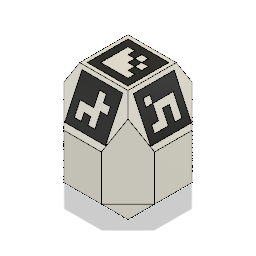
Tracking_die_smaller (Autodesk Fusion 360 design; units mm, degrees)
Autodesk Fusion 360 part; units mm, degrees
note: some values were not read from the file. Set by a fixed rule: which sketch regions a step uses; which face or edge a step refers to.
sketch "Sketch1" plane through (0, 0, 0) normal (0, 1, 0) x (1, 0, 0)
  line L0 (10, -10) -> (-10, -10)
  line L1 (-10, -10) -> (-10, 10)
  line L2 (-10, 10) -> (10, 10)
  line L3 (10, 10) -> (10, -10)
  line L4 (10, -10) -> (-10, 10) construction
  line L5 (-10, -10) -> (10, 10) construction
  dimension "d1" = 20
  dimension "d2" = 20
  constraint perpendicular L0 L1
  constraint parallel L0 L2
  constraint parallel L1 L3
  constraint horizontal L0
  constraint coincident L4 origin
  constraint coincident L5 origin
  measures "d1" distance of L0.end L1.end
  measures "d2" distance of L1.end L2.end
sketch "Sketch3" plane through (0, 0, 0) normal (0, 1, 0) x (1, 0, 0)
  line L0 (10, 10) -> (-10, 10)
  line L1 (-10, 10) -> (-10, -10)
  line L2 (-10, -10) -> (10, -10)
  line L3 (10, -10) -> (10, 10)
  line L4 (10, 10) -> (-10, -10) construction
  line L5 (-10, 10) -> (10, -10) construction
  dimension "d9" = 20
  dimension "d10" = 20
  constraint perpendicular L0 L1
  constraint parallel L0 L2
  constraint parallel L1 L3
  constraint horizontal L0
  constraint coincident L4 origin
  constraint coincident L5 origin
  measures "d9" distance of L1.end L2.end
  measures "d10" distance of L0.end L1.end
extrude "Extrude1" add sketch "Sketch1" along normal blind 10 makes body 1
sketch "Sketch2" plane through (0, 0, 0) normal (0, 1, 0) x (1, 0, 0)
  line L0 (14.1421, 0) -> (0, -14.1421)
  line L1 (0, -14.1421) -> (-14.1421, 0)
  line L2 (-14.1421, 0) -> (0, 14.1421)
  line L3 (0, 14.1421) -> (14.1421, 0)
  line L4 (14.1421, 0) -> (-14.1421, 0) construction
  line L5 (0, -14.1421) -> (0, 14.1421) construction
  dimension "d5" = 20
  dimension "d6" = 20
  constraint perpendicular L0 L1
  constraint parallel L0 L2
  constraint parallel L1 L3
  constraint coincident L4 origin
  constraint coincident L5 origin
  measures "d5" distance of L1.end L2.end
  measures "d6" distance of L0.end L1.end
sketch "Sketch4" plane through (0, 10, 0) normal (0, 1, 0) x (-1, 0, 0)
  line L0 (-10, -10) -> (10, -10)
  line L1 (10, -10) -> (10, 10)
  line L2 (10, 10) -> (-10, 10)
  line L3 (-10, 10) -> (-10, -10)
  line L4 (-10, -10) -> (10, -10)
  line L5 (10, -10) -> (10, 10)
  line L6 (10, 10) -> (-10, 10)
  line L7 (-10, 10) -> (-10, -10)
  line L8 (-10, -10) -> (10, 10) construction
  line L9 (10, -10) -> (-10, 10) construction
  dimension "d11" = 20
  dimension "d12" = 20
  constraint perpendicular L4 L5
  constraint parallel L4 L6
  constraint parallel L5 L7
  constraint horizontal L4
  constraint coincident L8 origin
  constraint coincident L9 origin
  measures "d11" distance of L1.end L2.end
  measures "d12" distance of L0.end L1.end
extrude "Extrude3" add sketch "Sketch4" along normal blind 10 draft -25 bodies 1
move_body "Move1" bodies 1 to x (1, 0, 0) y (0, 1, 0) z (0, 0, 1) at (0, 5, 0)
sketch "Sketch5" plane through (0, 5, 0) normal (0, -1, 0) x (1, 0, 0)
  line L0 (-10, -10) -> (10, -10)
  line L1 (10, -10) -> (10, 10)
  line L2 (10, 10) -> (-10, 10)
  line L3 (-10, 10) -> (-10, -10)
  line L4 (10, -10) -> (-10, -10)
  line L5 (-10, -10) -> (-10, 10)
  line L6 (-10, 10) -> (10, 10)
  line L7 (10, 10) -> (10, -10)
  line L8 (10, -10) -> (-10, 10) construction
  line L9 (-10, -10) -> (10, 10) construction
  dimension "d15" = 20
  dimension "d16" = 20
  constraint perpendicular L4 L5
  constraint parallel L4 L6
  constraint parallel L5 L7
  constraint horizontal L4
  constraint coincident L8 origin
  constraint coincident L9 origin
  measures "d15" distance of L2.end L1.end
  measures "d16" distance of L0.start L2.end
extrude "Extrude4" add sketch "Sketch3" against normal blind 5 draft -45 separate body makes body 2
move_body "Move2" bodies 1 to x (1, 0, 0) y (0, 1, 0) z (0, 0, 1) at (0, -5, 0)
sketch "Sketch6" plane through (0, 20, 0) normal (0, 1, 0) x (-1, 0, 0)
  line L0 (5.3369, 5.3369) -> (-5.3369, 5.3369)
  line L1 (-5.3369, 5.3369) -> (-5.3369, -5.3369)
  line L2 (-5.3369, -5.3369) -> (5.3369, -5.3369)
  line L3 (5.3369, -5.3369) -> (5.3369, 5.3369)
  line L4 (-14.1421, 0) -> (0, 14.1421)
  line L5 (0, 14.1421) -> (14.1421, 0)
  line L6 (14.1421, 0) -> (0, -14.1421)
  line L7 (0, -14.1421) -> (-14.1421, 0)
  line L8 (-14.1421, 0) -> (14.1421, 0) construction
  line L9 (0, 14.1421) -> (0, -14.1421) construction
  line L10 (-15.1463, -15.1463) -> (15.1463, -15.1463)
  line L11 (15.1463, -15.1463) -> (15.1463, 15.1463)
  line L12 (15.1463, 15.1463) -> (-15.1463, 15.1463)
  line L13 (-15.1463, 15.1463) -> (-15.1463, -15.1463)
  line L14 (-15.1463, -15.1463) -> (15.1463, 15.1463) construction
  line L15 (15.1463, -15.1463) -> (-15.1463, 15.1463) construction
  dimension "d19" = 20
  dimension "d20" = 20
  constraint perpendicular L4 L5
  constraint parallel L4 L6
  constraint parallel L5 L7
  constraint coincident L8 origin
  constraint coincident L9 origin
  constraint perpendicular L10 L11
  constraint parallel L10 L12
  constraint parallel L11 L13
  constraint horizontal L10
  constraint coincident L14 origin
  constraint coincident L15 origin
  measures "d19" distance of L5.end L6.end
  measures "d20" distance of L4.end L5.end
extrude "Extrude5" cut sketch "Sketch6" against normal blind 25 contours L10 L11 L12 L13 bodies 1 2
sketch "Sketch23" plane through (0, -5, 0) normal (0, -1, 0) x (1, 0, 0)
  line L0 (-5, -5) -> (5, -5)
  line L1 (5, -5) -> (5, 5)
  line L2 (5, 5) -> (-5, 5)
  line L3 (-5, 5) -> (-5, -5)
  line L4 (3.5183, 5.5393) -> (-5.5622, -3.482)
  line L5 (-5.5622, -3.482) -> (-3.5183, -5.5393)
  line L6 (-3.5183, -5.5393) -> (5.5622, 3.482)
  line L7 (5.5622, 3.482) -> (3.5183, 5.5393)
  line L8 (3.5183, 5.5393) -> (-3.5183, -5.5393) construction
  line L9 (-5.5622, -3.482) -> (5.5622, 3.482) construction
  dimension "d418" = 12.8
  dimension "d419" = 2.9
  constraint perpendicular L4 L5
  constraint parallel L4 L6
  constraint parallel L5 L7
  constraint coincident L8 origin
  constraint coincident L9 origin
  measures "d418" distance of L5.end L6.end
  measures "d419" distance of L4.end L5.end
sketch "Sketch8" plane through (-12.0442, 5.6163, 0) normal (-0.906308, 0.422618, 0) x (0, 0, 1)
  line L0 (4.1421, 4.8369) -> (7.0711, 11.7673)
  line L1 (7.0711, 11.7673) -> (5.3369, 15.8707)
  line L2 (5.3369, 15.8707) -> (-5.3369, 15.8707)
  line L3 (-5.3369, 15.8707) -> (-7.0711, 11.7673)
  line L4 (-7.0711, 11.7673) -> (-4.1421, 4.8369)
  line L5 (-4.1421, 4.8369) -> (4.1421, 4.8369)
  line L6 (-4.5277, 15.1063) -> (4.4723, 15.1063)
  line L7 (4.4723, 15.1063) -> (4.4723, 6.1063)
  line L8 (4.4723, 6.1063) -> (-4.5277, 6.1063)
  line L9 (-4.5277, 6.1063) -> (-4.5277, 15.1063)
  line L10 (-4.5277, 13.6063) -> (-4.5277, 12.1063)
  line L11 (-4.5277, 12.1063) -> (-4.5277, 10.6063)
  line L12 (-4.5277, 10.6063) -> (-4.5437, 9.1064)
  line L13 (-4.5437, 9.1064) -> (-4.553, 7.6064)
  line L14 (-4.553, 7.6064) -> (-4.5277, 6.1063)
  line L15 (-3.0277, 15.1063) -> (-1.5277, 15.1063)
  line L16 (-1.5277, 15.1063) -> (-0.0277, 15.1063)
  line L17 (-0.0277, 15.1063) -> (1.4723, 15.1063)
  line L18 (1.4723, 15.1063) -> (2.9723, 15.1063)
  line L19 (2.9814, 13.6063) -> (1.4814, 13.6063)
  line L20 (1.4814, 13.6063) -> (1.4814, 12.1063)
  line L21 (1.4814, 12.1063) -> (2.9814, 12.1063)
  line L22 (2.9814, 12.1063) -> (2.9814, 13.6063)
  line L23 (1.4814, 12.1063) -> (-0.0186, 12.1063)
  line L24 (-0.0186, 12.1063) -> (-0.0186, 10.6063)
  line L25 (-0.0186, 10.6063) -> (1.4814, 10.6063)
  line L26 (1.4814, 10.6063) -> (1.4814, 12.1063)
  line L27 (1.4814, 10.6063) -> (1.4814, 9.1063)
  line L28 (1.4814, 10.6063) -> (2.9814, 10.6063)
  line L29 (2.9814, 10.6063) -> (2.9814, 7.6063)
  line L30 (2.9814, 7.6063) -> (-1.5186, 7.6063)
  line L31 (-1.5186, 7.6063) -> (-1.5186, 9.1063)
  line L32 (1.4814, 9.1063) -> (-0.0186, 9.1063)
  line L33 (-0.0186, 9.1063) -> (-0.0186, 10.6063)
  line L34 (-0.0186, 10.6063) -> (-3.0186, 10.6063)
  line L35 (-3.0186, 10.6063) -> (-3.0186, 9.1063)
  line L36 (-3.0186, 9.1063) -> (-1.5186, 9.1063)
  dimension "d27" = 9
  dimension "d28" = 9
  dimension "d31" = 1.5
  dimension "d32" = 1.5
  dimension "d33" = 1.5
  dimension "d34" = 1.5
  dimension "d35" = 1.5
  dimension "d36" = 1.5
  dimension "d37" = 1.5
  dimension "d38" = 1.5
  dimension "d317" = 1.5
  dimension "d318" = 1.5
  dimension "d319" = 1.5
  dimension "d320" = 1.5
  dimension "d329" = 1.5
  dimension "d330" = 1.5
  dimension "d331" = 3
  dimension "d332" = 4.5
  dimension "d333" = 1.5
  dimension "d334" = 1.5
  dimension "d335" = 3
  dimension "d336" = 1.5
  constraint horizontal L6
  constraint vertical L7
  constraint horizontal L8
  constraint vertical L9
  constraint coincident L9 L10.start
  constraint coincident L6 L15.start
  constraint midpoint L9 L11.end
  constraint parallel L6 L16
  constraint parallel L6 L17
  constraint parallel L6 L18
  constraint horizontal L19
  constraint vertical L20
  constraint horizontal L21
  constraint vertical L22
  constraint horizontal L23
  constraint vertical L24
  constraint horizontal L25
  constraint vertical L26
  constraint perpendicular L25 L27
  constraint perpendicular L27 L28
  constraint perpendicular L28 L29
  constraint perpendicular L29 L30
  constraint perpendicular L30 L31
  constraint perpendicular L27 L32
  constraint perpendicular L24 L34
  constraint perpendicular L34 L35
  measures "d27" distance of L6.start L6.end
  measures "d28" distance of L6.start L8.end
  measures "d31" distance of L10.start L10.end
  measures "d32" distance of L10.end L11.end
  measures "d33" distance of L11.end L12.end
  measures "d34" distance of L12.end L13.end
  measures "d35" distance of L15.start L15.end
  measures "d36" distance of L15.end L16.end
  measures "d37" distance of L16.end L17.end
  measures "d38" distance of L17.end L18.end
  measures "d317" distance of L19.start L19.end
  measures "d318" distance of L19.start L21.end
  measures "d319" distance of L20.end L23.end
  measures "d320" distance of L20.end L25.end
  measures "d329" distance of L25.end L27.end
  measures "d330" distance of L25.end L28.end
  measures "d331" distance of L28.end L29.end
  measures "d332" distance of L29.end L30.end
  measures "d333" distance of L30.end L31.end
  measures "d334" distance of L27.end L32.end
  measures "d335" distance of L24.end L34.end
  measures "d336" distance of L34.end L35.end
sketch "Sketch13" plane through (0, 5.6163, -12.0442) normal (0, 0.422618, -0.906308) x (-1, 0, 0)
  line L0 (-7.0711, 11.7673) -> (-4.1421, 4.8369)
  line L1 (-4.1421, 4.8369) -> (4.1421, 4.8369)
  line L2 (4.1421, 4.8369) -> (7.0711, 11.7673)
  line L3 (7.0711, 11.7673) -> (5.3369, 15.8707)
  line L4 (5.3369, 15.8707) -> (-5.3369, 15.8707)
  line L5 (-5.3369, 15.8707) -> (-7.0711, 11.7673)
  line L6 (-4.5, 15) -> (4.5, 15)
  line L7 (4.5, 15) -> (4.5, 6)
  line L8 (4.5, 6) -> (-4.5, 6)
  line L9 (-4.5, 6) -> (-4.5, 15)
  line L10 (-4.5, 15) -> (-4.5, 13.5)
  line L11 (-4.5, 13.5) -> (-4.5, 12)
  line L12 (-4.5, 12) -> (-4.5, 10.5)
  line L13 (-4.5, 10.5) -> (-4.5, 12)
  line L14 (-4.5, 12) -> (-4.5, 10.5)
  line L15 (-4.5, 6) -> (-4.5, 10.5)
  line L16 (-4.5, 15) -> (-3, 15)
  line L17 (-3, 15) -> (-1.5, 15)
  line L18 (-1.5, 15) -> (0, 15)
  line L19 (0, 15) -> (1.5, 15)
  line L20 (1.5, 15) -> (3, 15)
  line L21 (-3, 7.5) -> (-3, 10.5)
  line L22 (-3, 10.5) -> (-1.5, 10.5)
  line L23 (-1.5, 10.5) -> (-1.5, 9)
  line L24 (-1.5, 9) -> (1.5, 9)
  line L25 (1.5, 9) -> (1.5, 10.5)
  line L26 (3, 10.5) -> (3, 9)
  line L27 (3, 9) -> (1.5, 9)
  line L28 (1.5, 9) -> (1.5, 7.5)
  line L29 (1.5, 12) -> (3, 12)
  line L30 (1.5, 12) -> (1.5, 13.5)
  line L31 (3, 12) -> (3, 13.5)
  line L32 (1.5, 13.5) -> (3, 13.5)
  line L33 (-3, 7.5) -> (1.5, 7.5)
  line L34 (-1.5, 10.5) -> (0, 10.5)
  line L35 (0, 10.5) -> (0, 12)
  line L36 (-1.5, 10.5) -> (-1.5, 13.5)
  line L37 (0, 10.5) -> (0, 13.5)
  line L38 (-1.5, 13.5) -> (0, 13.5)
  line L39 (1.5, 10.5) -> (3, 10.5)
  dimension "d39" = 9
  dimension "d40" = 9
  dimension "d41" = 1.5
  dimension "d42" = 1.5
  dimension "d43" = 1.5
  dimension "d44" = 1.5
  dimension "d45" = 1.5
  dimension "d46" = 1.5
  dimension "d47" = 1.5
  dimension "d48" = 1.5
  dimension "d49" = 1.5
  dimension "d341" = 3
  dimension "d342" = 1.5
  dimension "d343" = 1.5
  dimension "d344" = 3
  dimension "d345" = 1.5
  dimension "d346" = 3
  dimension "d347" = 3
  constraint horizontal L6
  constraint vertical L7
  constraint horizontal L8
  constraint vertical L9
  constraint coincident L6 L16.end
  constraint perpendicular L6 L10
  constraint coincident L9 L11.end
  constraint midpoint L9 L12.end
  constraint parallel L9 L14
  constraint midpoint L6 L18.end
  constraint parallel L6 L19
  constraint coincident L6 L20.end
  constraint perpendicular L21 L22
  constraint perpendicular L22 L23
  constraint perpendicular L23 L24
  constraint perpendicular L24 L25
  constraint perpendicular L28 L33
  constraint perpendicular L23 L34
  constraint perpendicular L22 L35
  constraint perpendicular L34 L36
  constraint perpendicular L34 L37
  constraint perpendicular L37 L38
  constraint perpendicular L26 L39
  measures "d39" distance of L6.start L6.end
  measures "d40" distance of L6.start L8.end
  measures "d41" distance of L6.start L10.end
  measures "d42" distance of L10.end L11.end
  measures "d43" distance of L11.end L12.end
  measures "d44" distance of L12.end L11.end
  measures "d45" distance of L11.end L12.end
  measures "d46" distance of L16.end L17.end
  measures "d47" distance of L17.end L18.end
  measures "d48" distance of L18.end L19.end
  measures "d49" distance of L19.end L20.end
  measures "d341" distance of L21.start L21.end
  measures "d342" distance of L21.end L22.end
  measures "d343" distance of L22.end L23.end
  measures "d344" distance of L23.end L24.end
  measures "d345" distance of L24.end L25.end
  measures "d346" distance of L22.end L36.end
  measures "d347" distance of L34.end L37.end
sketch "Sketch14" plane through (12.0442, 5.6163, 0) normal (0.906308, 0.422618, 0) x (0, 0, -1)
  line L0 (4.1421, 4.8369) -> (7.0711, 11.7673)
  line L1 (7.0711, 11.7673) -> (5.3369, 15.8707)
  line L2 (5.3369, 15.8707) -> (-5.3369, 15.8707)
  line L3 (-5.3369, 15.8707) -> (-7.0711, 11.7673)
  line L4 (-7.0711, 11.7673) -> (-4.1421, 4.8369)
  line L5 (-4.1421, 4.8369) -> (4.1421, 4.8369)
  line L6 (-4.5281, 14.9652) -> (4.4719, 14.9652)
  line L7 (4.4719, 14.9652) -> (4.4719, 5.9652)
  line L8 (4.4719, 5.9652) -> (-4.5281, 5.9652)
  line L9 (-4.5281, 5.9652) -> (-4.5281, 14.9652)
  line L10 (-4.5281, 14.9652) -> (-3.0281, 14.9652)
  line L11 (-3.0281, 14.9652) -> (-1.5281, 14.9652)
  line L12 (-1.5281, 14.9652) -> (-0.0281, 14.9652)
  line L13 (-0.0281, 14.9652) -> (1.4719, 14.9652)
  line L14 (1.4719, 14.9652) -> (2.9719, 14.9652)
  line L15 (-4.5281, 14.9652) -> (-4.5281, 13.4566)
  line L16 (-4.5281, 14.9652) -> (-4.5281, 13.4652)
  line L17 (-4.5281, 13.4566) -> (-4.5281, 11.9566)
  line L18 (-4.5281, 11.9566) -> (-4.5281, 10.4566)
  line L19 (-4.5281, 10.4566) -> (-4.5281, 8.9566)
  line L20 (-4.5281, 8.9566) -> (-4.5281, 7.4566)
  line L21 (-3.0281, 7.4566) -> (-0.0281, 7.4566)
  line L22 (-0.0281, 7.4566) -> (-0.0281, 10.4566)
  line L23 (-0.0281, 10.4566) -> (1.4719, 10.4566)
  line L24 (1.4719, 10.4566) -> (1.4719, 7.4566)
  line L25 (1.4719, 7.4566) -> (2.9719, 7.4566)
  line L26 (2.9719, 7.4566) -> (2.9719, 11.9566)
  line L27 (2.9719, 11.9566) -> (-1.5281, 11.9566)
  line L28 (-1.5281, 11.9566) -> (-1.5281, 8.9566)
  line L29 (-1.5281, 8.9566) -> (-3.0281, 8.9566)
  line L30 (-3.0281, 8.9566) -> (-3.0281, 7.4566)
  line L31 (-1.5281, 11.9566) -> (-1.5281, 13.4566)
  line L32 (-1.5281, 13.4566) -> (-3.0281, 13.4566)
  line L33 (-3.0281, 13.4566) -> (-3.0281, 11.9566)
  line L34 (-3.0281, 11.9566) -> (-1.5281, 11.9566)
  dimension "d50" = 9
  dimension "d51" = 9
  dimension "d52" = 1.5
  dimension "d53" = 1.5
  dimension "d54" = 1.5
  dimension "d55" = 1.5
  dimension "d56" = 1.5
  dimension "d57" = 1.5
  dimension "d58" = 1.5
  dimension "d59" = 1.5
  dimension "d60" = 1.5
  dimension "d61" = 1.5
  dimension "d352" = 3
  dimension "d353" = 3
  dimension "d354" = 1.5
  dimension "d355" = 1.5
  dimension "d356" = 4.5
  dimension "d357" = 4.5
  dimension "d358" = 3
  dimension "d359" = 1.5
  dimension "d360" = 1.5
  dimension "d361" = 1.5
  dimension "d362" = 1.5
  dimension "d363" = 1.5
  constraint horizontal L6
  constraint vertical L7
  constraint horizontal L8
  constraint vertical L9
  constraint perpendicular L9 L10
  constraint perpendicular L9 L11
  constraint parallel L6 L12
  constraint parallel L6 L13
  constraint parallel L6 L14
  constraint coincident L9 L15.end
  constraint perpendicular L6 L16
  constraint parallel L9 L17
  constraint parallel L9 L18
  constraint parallel L9 L19
  constraint parallel L9 L20
  constraint perpendicular L22 L23
  constraint perpendicular L25 L26
  constraint perpendicular L26 L27
  constraint perpendicular L27 L28
  constraint perpendicular L28 L29
  constraint perpendicular L21 L30
  constraint perpendicular L27 L31
  constraint perpendicular L31 L32
  constraint perpendicular L32 L33
  measures "d50" distance of L6.start L6.end
  measures "d51" distance of L6.start L8.end
  measures "d52" distance of L6.start L10.end
  measures "d53" distance of L10.end L11.end
  measures "d54" distance of L11.end L12.end
  measures "d55" distance of L12.end L13.end
  measures "d56" distance of L13.end L14.end
  measures "d57" distance of L6.start L16.end
  measures "d58" distance of L15.end L17.end
  measures "d59" distance of L17.end L18.end
  measures "d60" distance of L18.end L19.end
  measures "d61" distance of L19.end L20.end
  measures "d352" distance of L21.start L21.end
  measures "d353" distance of L21.end L22.end
  measures "d354" distance of L22.end L23.end
  measures "d355" distance of L24.end L25.end
  measures "d356" distance of L25.end L26.end
  measures "d357" distance of L26.end L27.end
  measures "d358" distance of L27.end L28.end
  measures "d359" distance of L28.end L29.end
  measures "d360" distance of L29.end L21.start
  measures "d361" distance of L27.end L31.end
  measures "d362" distance of L31.end L32.end
  measures "d363" distance of L32.end L33.end
sketch "Sketch15" plane through (0, 5.6163, 12.0442) normal (0, 0.422618, 0.906308) x (1, 0, 0)
  line L0 (4.1421, 4.8369) -> (7.0711, 11.7673)
  line L1 (7.0711, 11.7673) -> (5.3369, 15.8707)
  line L2 (5.3369, 15.8707) -> (-5.3369, 15.8707)
  line L3 (-5.3369, 15.8707) -> (-7.0711, 11.7673)
  line L4 (-7.0711, 11.7673) -> (-4.1421, 4.8369)
  line L5 (-4.1421, 4.8369) -> (4.1421, 4.8369)
  line L6 (-4.4601, 15.0583) -> (4.5399, 15.0583)
  line L7 (4.5399, 15.0583) -> (4.5399, 6.0583)
  line L8 (4.5399, 6.0583) -> (-4.4601, 6.0583)
  line L9 (-4.4601, 6.0583) -> (-4.4601, 15.0583)
  line L10 (-4.4601, 15.0583) -> (-2.9601, 15.0583)
  line L11 (-2.9601, 15.0583) -> (-1.3135, 15.0583)
  line L12 (-2.9601, 15.0583) -> (-1.4601, 15.0583)
  line L13 (-1.4601, 15.0583) -> (0.0399, 15.0583)
  line L14 (0.0399, 15.0583) -> (1.5399, 15.0583)
  line L15 (1.5399, 15.0583) -> (3.0399, 15.0583)
  line L16 (-4.4601, 15.0583) -> (-4.4601, 13.5583)
  line L17 (-4.4601, 13.5583) -> (-4.4601, 12.0583)
  line L18 (-4.4601, 12.0583) -> (-4.4601, 10.5583)
  line L19 (-4.4601, 10.5583) -> (-4.4601, 9.0583)
  line L20 (-4.4601, 9.0583) -> (-4.4601, 7.5583)
  line L21 (-2.9601, 7.5583) -> (-1.4601, 7.5583)
  line L22 (-2.9601, 7.5583) -> (-2.9601, 10.5583)
  line L23 (-2.9601, 10.5583) -> (0.0399, 10.5583)
  line L24 (-1.4601, 7.5583) -> (-1.4601, 9.0583)
  line L25 (-1.4601, 9.0583) -> (0.0399, 9.0583)
  line L26 (0.0399, 9.0583) -> (0.0399, 7.5583)
  line L27 (0.0399, 7.5583) -> (1.5399, 7.5583)
  line L28 (1.5399, 7.5583) -> (1.5399, 10.5583)
  line L29 (1.5399, 10.5583) -> (3.0399, 10.5583)
  line L30 (3.0399, 10.5583) -> (3.0399, 12.0583)
  line L31 (3.0399, 12.0583) -> (1.5399, 12.0583)
  line L32 (1.5399, 12.0583) -> (1.5399, 13.5583)
  line L33 (1.5399, 13.5583) -> (0.0399, 13.5583)
  line L34 (0.0399, 13.5583) -> (0.0399, 10.5583)
  dimension "d62" = 9
  dimension "d63" = 9
  dimension "d64" = 1.5
  dimension "d65" = 1.5
  dimension "d66" = 1.5
  dimension "d67" = 1.5
  dimension "d68" = 1.5
  dimension "d69" = 1.5
  dimension "d70" = 1.5
  dimension "d71" = 1.5
  dimension "d72" = 1.5
  dimension "d73" = 1.5
  dimension "d368" = 1.5
  dimension "d369" = 3
  dimension "d370" = 3
  dimension "d371" = 1.5
  dimension "d372" = 1.5
  dimension "d373" = 1.5
  dimension "d374" = 3
  dimension "d375" = 1.5
  dimension "d376" = 1.5
  dimension "d377" = 1.5
  dimension "d378" = 1.5
  dimension "d379" = 1.5
  dimension "d380" = 3
  constraint horizontal L6
  constraint vertical L7
  constraint horizontal L8
  constraint vertical L9
  constraint perpendicular L9 L10
  constraint coincident L6 L11.end
  constraint parallel L6 L12
  constraint midpoint L6 L13.end
  constraint parallel L6 L14
  constraint parallel L6 L15
  constraint perpendicular L10 L16
  constraint parallel L9 L17
  constraint parallel L9 L18
  constraint parallel L9 L19
  constraint parallel L9 L20
  constraint perpendicular L24 L25
  constraint perpendicular L25 L26
  constraint perpendicular L24 L27
  constraint perpendicular L27 L28
  constraint perpendicular L28 L29
  constraint perpendicular L29 L30
  constraint perpendicular L30 L31
  constraint perpendicular L32 L33
  measures "d62" distance of L6.start L6.end
  measures "d63" distance of L6.start L8.end
  measures "d64" distance of L6.start L10.end
  measures "d65" distance of L10.end L12.end
  measures "d66" distance of L12.end L13.end
  measures "d67" distance of L13.end L14.end
  measures "d68" distance of L14.end L15.end
  measures "d69" distance of L6.start L16.end
  measures "d70" distance of L16.end L17.end
  measures "d71" distance of L17.end L18.end
  measures "d72" distance of L18.end L19.end
  measures "d73" distance of L19.end L20.end
  measures "d368" distance of L21.start L21.end
  measures "d369" distance of L21.start L22.end
  measures "d370" distance of L22.end L23.end
  measures "d371" distance of L21.end L24.end
  measures "d372" distance of L24.end L25.end
  measures "d373" distance of L26.end L27.end
  measures "d374" distance of L27.end L28.end
  measures "d375" distance of L28.end L29.end
  measures "d376" distance of L29.end L30.end
  measures "d377" distance of L30.end L31.end
  measures "d378" distance of L31.end L32.end
  measures "d379" distance of L32.end L33.end
  measures "d380" distance of L33.end L23.end
sketch "Sketch16" plane through (0, 20, 0) normal (0, 1, 0) x (-1, 0, 0)
  line L0 (5.3369, 5.3369) -> (-5.3369, 5.3369)
  line L1 (-5.3369, 5.3369) -> (-5.3369, -5.3369)
  line L2 (-5.3369, -5.3369) -> (5.3369, -5.3369)
  line L3 (5.3369, -5.3369) -> (5.3369, 5.3369)
  line L4 (4.5, -4.5) -> (-4.5, -4.5)
  line L5 (-4.5, -4.5) -> (-4.5, 4.5)
  line L6 (-4.5, 4.5) -> (4.5, 4.5)
  line L7 (4.5, 4.5) -> (4.5, -4.5)
  line L8 (4.5, -4.5) -> (3, -4.5)
  line L9 (4.5, -4.5) -> (4.5, -3)
  line L10 (4.5, -3) -> (4.5, -1.5)
  line L11 (4.5, -1.5) -> (4.5, 0)
  line L12 (4.5, 0) -> (4.5, 1.6193)
  line L13 (4.5, 0) -> (4.5, 1.5)
  line L14 (4.5, 1.5) -> (4.5, 3)
  line L15 (4.5, -4.5) -> (3, -4.5)
  line L16 (3, -4.5) -> (1.5, -4.5)
  line L17 (1.5, -4.5) -> (0, -4.5)
  line L18 (0, -4.5) -> (-1.5, -4.5)
  line L19 (-1.5, -4.5) -> (-3, -4.5)
  line L20 (-3, -4.5) -> (-1.5, -4.5)
  line L21 (3, -3) -> (1.5, -3)
  line L22 (1.5, -3) -> (1.5, -1.5)
  line L23 (1.5, -1.5) -> (0, -1.5)
  line L24 (0, -1.5) -> (0, 0)
  line L25 (0, -1.5) -> (0, -3)
  line L26 (0, -1.5) -> (-1.5, -1.5)
  line L27 (-1.5, -1.5) -> (-1.5, -3)
  line L28 (-1.5, -3) -> (0, -3)
  line L29 (3, -3) -> (3, 3)
  line L30 (3, 3) -> (-3, 3)
  line L31 (-3, 3) -> (-3, 1.5)
  line L32 (-3, 1.5) -> (-1.5, 1.5)
  line L33 (-1.5, 1.5) -> (-1.5, 0)
  line L34 (-1.5, 0) -> (0, 0)
  line L35 (-1.5, -1.5) -> (-1.5, 0)
  line L36 (-1.5, 0) -> (-3, 0)
  line L37 (-3, 0) -> (-3, -1.5)
  line L38 (-3, -1.5) -> (-1.5, -1.5)
  dimension "d74" = 9
  dimension "d75" = 9
  dimension "d76" = 1.5
  dimension "d77" = 1.5
  dimension "d78" = 1.5
  dimension "d79" = 1.5
  dimension "d80" = 1.5
  dimension "d81" = 1.5
  dimension "d82" = 1.5
  dimension "d83" = 1.5
  dimension "d84" = 1.5
  dimension "d85" = 1.5
  dimension "d385" = 1.5
  dimension "d386" = 1.5
  dimension "d387" = 1.5
  dimension "d388" = 1.5
  dimension "d392" = 6
  dimension "d393" = 6
  dimension "d394" = 1.5
  dimension "d395" = 1.5
  dimension "d396" = 1.5
  dimension "d397" = 1.5
  dimension "d398" = 1.5
  constraint perpendicular L4 L5
  constraint parallel L4 L6
  constraint parallel L5 L7
  constraint horizontal L4
  constraint coincident L24.end L34.end
  constraint coincident L4 L8.end
  constraint perpendicular L3 L8
  constraint perpendicular L8 L9
  constraint parallel L7 L10
  constraint midpoint L7 L11.end
  constraint coincident L7 L12.end
  constraint parallel L12 L13
  constraint coincident L7 L14.end
  constraint parallel L4 L16
  constraint midpoint L4 L17.end
  constraint parallel L4 L18
  constraint coincident L4 L19.end
  constraint parallel L4 L19
  constraint vertical L22
  constraint perpendicular L22 L23
  constraint perpendicular L23 L24
  constraint perpendicular L25 L26
  constraint perpendicular L21 L29
  constraint perpendicular L29 L30
  constraint perpendicular L30 L31
  constraint perpendicular L31 L32
  constraint perpendicular L32 L33
  constraint perpendicular L33 L36
  constraint perpendicular L26 L37
  measures "d74" distance of L5.end L6.end
  measures "d75" distance of L4.end L5.end
  measures "d76" distance of L4.start L9.end
  measures "d77" distance of L9.end L10.end
  measures "d78" distance of L10.end L11.end
  measures "d79" distance of L11.end L13.end
  measures "d80" distance of L13.end L14.end
  measures "d81" distance of L4.start L8.end
  measures "d82" distance of L8.end L16.end
  measures "d83" distance of L16.end L17.end
  measures "d84" distance of L17.end L18.end
  measures "d85" distance of L18.end L19.end
  measures "d385" distance of L21.start L21.end
  measures "d386" distance of L21.end L22.end
  measures "d387" distance of L22.end L23.end
  measures "d388" distance of L23.end L24.end
  measures "d392" distance of L21.start L29.end
  measures "d393" distance of L29.end L30.end
  measures "d394" distance of L30.end L31.end
  measures "d395" distance of L31.end L32.end
  measures "d396" distance of L32.end L33.end
  measures "d397" distance of L33.end L36.end
  measures "d398" distance of L36.end L37.end
sketch "Sketch21" plane through (-7.0711, 0, 7.0711) normal (-0.707107, 0, 0.707107) x (0.707107, 0, 0.707107)
  line L0 (4.1421, 10) -> (0, 16.2811)
  line L1 (0, 16.2811) -> (-4.1421, 10)
  line L2 (-4.1421, 10) -> (-4.1421, 0)
  line L3 (-4.1421, 0) -> (4.1421, 0)
  line L4 (4.1421, 0) -> (4.1421, 10)
  circle A0 centre (0, 1) radius 3
  circle A1 centre (0, 1) radius 1.5
  dimension "d408" = 6
  dimension "d428" = 3
  constraint concentric A0 A1
  measures "d408" diameter of A0
  measures "d428" diameter of A1
extrude "Extrude103" cut sketch "Sketch23" against normal blind 23 contours L0 L1 L2 L3 L4 L5 L6 L7 | L0 L5 L6 | L3 L4 L5 | L1 L6 L7 | L2 L4 L7 bodies 1 2
sketch "Sketch24" plane through (7.0711, 0, -7.0711) normal (0.707107, 0, -0.707107) x (-0.707107, 0, -0.707107)
  line L0 (4.1421, 10) -> (0, 16.2811)
  line L1 (0, 16.2811) -> (-4.1421, 10)
  line L2 (-4.1421, 10) -> (-4.1421, 0)
  line L3 (-4.1421, 0) -> (4.1421, 0)
  line L4 (4.1421, 0) -> (4.1421, 10)
  circle A0 centre (0, 6) radius 1.5
  circle A1 centre (0, 6) radius 3
  dimension "d430" = 3
  dimension "d431" = 6
  constraint concentric A0 A1
  measures "d430" diameter of A0
  measures "d431" diameter of A1
extrude "Extrude107" cut sketch "Sketch24" against normal blind 20 contours A0 bodies 1
extrude "Extrude108" cut sketch "Sketch24" against normal blind 2.9 contours A1 bodies 1
extrude "Extrude109" cut sketch "Sketch21" against normal blind 20 contours L3 A1 picked at (0.4509, 0.5493) bodies 1
extrude "Extrude110" cut sketch "Sketch21" against normal blind 2.9 contours L3 A0 A1 picked at (-2.3736, 1.7678) bodies 1
extrude "Extrude111" cut sketch "Sketch21" against normal blind 20 contours L3 A1 picked at (0.3224, -0.0488) bodies 2
extrude "Extrude112" cut sketch "Sketch21" against normal blind 2.9 contours L3 A0 A1 picked at (0, -1.4948) bodies 2
extrude "Extrude93" cut sketch "Sketch8" against normal blind 0.3 contours L6 L7 L8 L9 L10 L11 L15 L16 L17 L18 | L25 L27 L32 L33 bodies 1
extrude "Extrude94" add 2 faces at (-6.4446, 16.9147, -2.5217) (-7.7125, 14.1958, 0.9814) along direction (-0.906308, 0.422618, 0) blind 0.3 separate body on bodies 1 makes body 3 at (-6.4446, 16.9147, -2.5217)
extrude "Extrude95" cut sketch "Sketch13" against normal blind 0.3 contours L6 L7 L8 L9 L10 L11 L12 L13 L14 L15 L16 L17 L18 L19 L20 bodies 1
extrude "Extrude96" add 1 faces at (3, 17.2715, -6.2782) along direction (0, 0.422618, -0.906308) blind 0.3 separate body on bodies 1 makes body 4
extrude "Extrude97" cut sketch "Sketch14" against normal blind 0.3 contours L6 L7 L8 L9 L10 L11 L12 L13 L14 L15 L16 L17 L18 L19 L20 bodies 1
extrude "Extrude98" add 1 faces at (6.084, 17.6879, -1.9719) along direction (0.906308, 0.422618, 0) blind 0.3 separate body on bodies 1 makes body 5
extrude "Extrude99" cut sketch "Sketch15" against normal blind 0.3 contours L6 L7 L8 L9 L10 L11 L12 L13 L14 L15 L16 L17 L18 L19 L20 bodies 1
extrude "Extrude100" add 1 faces at (-2.4601, 17.3244, 6.2536) along direction (0, 0.422618, 0.906308) blind 0.3 separate body on bodies 1 makes body 6
extrude "Extrude101" cut sketch "Sketch16" against normal blind 0.3 contours L4 L5 L6 L7 L8 L9 L10 L11 L12 L13 L14 L15 L16 L17 L18 L19 L20 | L24 L26 L34 L35 bodies 1
extrude "Extrude102" add 2 faces at (3, 19.7, -3) (0.5, 19.7, -1) along direction (0, 1, 0) blind 0.3 separate body on bodies 1 makes body 7 at (3, 19.7, -3)
